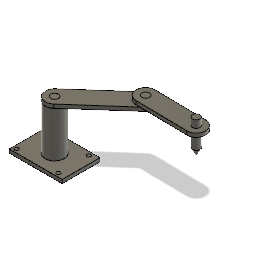
26-Day 20 - Robotic Arm v1 (Autodesk Fusion 360 design; units mm, degrees)
Autodesk Fusion 360 part; units mm, degrees
note: some values were not read from the file. Set by a fixed rule: which sketch regions a step uses.
sketch "Sketch1" plane through (0, 0, 0) normal (0, 1, 0) x (1, 0, 0)
  line L0 (-70, 50) -> (70, 50)
  line L1 (70, 50) -> (70, -50)
  line L2 (70, -50) -> (-70, -50)
  line L3 (-70, -50) -> (-70, 50)
  circle A0 centre (0, 0) radius 25
  circle A1 centre (-60, -40) radius 5
  circle A2 centre (-60, 40) radius 5
  circle A3 centre (50, 40) radius 5
  circle A4 centre (50, -40) radius 5
  line L4 (0, 0) -> (0, 25)
  line L5 (0, 25) -> (170, 25)
  line L6 (170, -25) -> (0, -25)
  arc A5 (170, -25) -> (170, 25) centre (170, 0) ccw
  arc A6 (170, 25) -> (170, -25) centre (170, 0) ccw
  line L7 (170, 0) -> (190.6182, -14.1383)
  line L8 (170, 0) -> (149.3818, 14.1383)
  line L9 (149.3818, 14.1383) -> (226.1734, 126.1254)
  line L10 (267.4098, 97.8489) -> (190.6182, -14.1383)
  arc A7 (267.4098, 97.8489) -> (226.1734, 126.1254) centre (246.7916, 111.9872) ccw
  arc A8 (226.1734, 126.1254) -> (267.4098, 97.8489) centre (246.7916, 111.9872) ccw
  circle A9 centre (246.7916, 111.9872) radius 10
  circle A10 centre (0, 0) radius 10
  circle A11 centre (170, 0) radius 10
  dimension "d1" = 50
  dimension "d2" = 10
  dimension "d4" = 50
  dimension "d5" = 20
  dimension "d28" = 20
  dimension "d29" = 20
  constraint horizontal L0
  constraint vertical L1
  constraint horizontal L2
  constraint vertical L3
  constraint coincident A0.centre L4.start
  constraint equal A1 A2
  constraint equal A1 A3
  constraint equal A1 A4
  constraint coincident A0 L4.end
  constraint vertical L4
  constraint tangent A0 L5
  constraint coincident A0 L6.end
  constraint tangent A0 L6
  constraint tangent L5 A5
  constraint coincident A5.centre A6.centre
  constraint coincident A5 L7.end
  constraint coincident A6 L8.end
  constraint parallel L7 L8
  constraint tangent A6 L9
  constraint tangent A5 L10
  constraint coincident A7.centre A8.centre
  constraint concentric A7 A9
  constraint concentric A0 A10
  constraint concentric A5 A11
  measures "d1" diameter of A0
  measures "d2" diameter of A1
  measures "d4" distance of L9.end L10.start
  measures "d5" diameter of A9
  measures "d28" diameter of A10
  measures "d29" diameter of A11
extrude "Extrude1" add sketch "Sketch1" against normal blind 10 contours L0 L1 L2 L3 A0 L5 L6 | L1 A0 L5 L6 | A0 | A10 makes body 1
extrude "Extrude2" add sketch "Sketch1" against normal blind 10 separate body contours A1 | A2 | A3 | A4 makes body 2 at (-55.0062, -6.6667, 40.2492) makes body 3 at (54.9938, -6.6667, 40.2492) makes body 4 at (-55.0062, -6.6667, -39.7508) makes body 5 at (54.9938, -6.6667, -39.7508)
extrude "Extrude3" add sketch "Sketch1" along normal blind 120 separate body contours A0 | A10 makes body 6
extrude "Extrude4" add sketch "Sketch1" along normal blind 10 from surface at 120 separate body contours L1 L5 L6 A6 L9 | L1 A0 L5 L6 | A0 | L5 A6 L9 | A5 A6 L7 L8 A11 | A5 A6 L7 L8 A11 | L7 L8 A11 | L7 L8 A11 | A10 makes body 7
extrude "Extrude5" add sketch "Sketch1" along normal blind 10 from surface at 130 separate body contours L5 A5 L9 L10 A8 | L5 A6 L9 | A5 A6 L7 L8 A11 | A5 A6 L7 L8 A11 | A7 A8 | L7 L8 A11 | L7 L8 A11 | A9 makes body 8
extrude "Extrude6" cut sketch "Sketch1" along normal blind 10 and the other way blind 30 from surface at 140 contours A9 bodies 8
extrude "Extrude7" add sketch "Sketch1" along normal blind 10 and the other way blind 80 from surface at 140 separate body contours A9 makes body 9
extrude "Extrude8" cut sketch "Sketch1" along normal blind 170 contours A10 bodies 7
extrude "Extrude9" cut sketch "Sketch1" along normal blind 180 contours L7 L8 A11 | L7 L8 A11 bodies 7 8
extrude "Extrude10" cut sketch "Sketch1" against normal blind 120 from surface at 120 contours A10 bodies 6
extrude "Extrude1'" add sketch "Sketch1" along normal blind 130 separate body contours A10 makes body 10 in component "Rod BH1"
extrude "Extrude1''" add sketch "Sketch1" along normal mid plane 20 from surface at 130 separate body contours L7 L8 A11 | L7 L8 A11 makes body 11 in component "Rod H1H2"
combine "Combine1" operation add target body 7 tool bodies 11
combine "Combine2" operation add target body 1 tool bodies 10
combine "Combine3" operation add target body 1 tool bodies 6
copy_body "Body->Comp2" bodies 1 removing the originals makes body 12 in component "Base"
copy_body "Body->Comp3" bodies 7 removing the originals makes body 13 in component "Arm1"
copy_body "Body->Comp4" bodies 8 removing the originals makes body 14 in component "Arm2"
copy_body "Body->Comp5" bodies 9 removing the originals makes body 15 in component "End Effector"
chamfer "Chamfer1" distance 10 distance2 20 1 edges at (237.4683, 60, -115.6033) measured on face at (249.6761, 60, -105.9975) on bodies 15 in component "End Effector"
component "Base" placed x (1, 0, 0) y (0, 1, 0) z (0, 0, 1) at (0, 0, 0)
component "Arm1" placed x (1, 0, 0) y (0, 1, 0) z (0, 0, 1) at (0, 0, 0)
component "Arm2" placed x (1, 0, 0) y (0, 1, 0) z (0, 0, 1) at (0, 0, 0)
component "End Effector" placed x (1, 0, 0) y (0, 1, 0) z (0, 0, 1) at (0, -10, 0)
